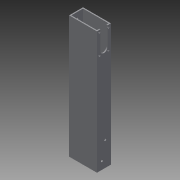
# Autodesk Inventor part: Arm_Second_Flame
Saved by Autodesk Inventor 2013 (Build 170138000, 138)
## iProperties
Created: 2014-04-16
Part Number: Arm_Second_Flame
Material: 一般
Document SubType Name: Modeling
Designer: andou
Density: 1 g/cm^3
Author: andou
Autodesk Inventor part; units mm, degrees
ref_plane "YZ Plane" through (0, 0, 0) normal (1, 0, 0) x (0, 1, 0)
ref_plane "XZ Plane" through (0, 0, 0) normal (0, 1, 0) x (-1, 0, 0)
ref_plane "XY Plane" through (0, 0, 0) normal (0, 0, 1) x (1, 0, 0)
sketch "スケッチ1" plane through (0, 0, 0) normal (0, 0, 1) x (1, 0, 0)
  line L0 (-25, 12.5) -> (25, 12.5)
  line L1 (25, 12.5) -> (25, -12.5)
  line L2 (25, -12.5) -> (-25, -12.5)
  line L3 (-25, -12.5) -> (-25, 12.5)
  line L4 (-23, 10.5) -> (23, 10.5)
  line L5 (23, 10.5) -> (23, -10.5)
  line L6 (23, -10.5) -> (-23, -10.5)
  line L7 (-23, -10.5) -> (-23, 10.5)
  point P0 (0, 0)
  dimension "d0" = 50
  dimension "d2" = 25
  dimension "d3" = 21
  dimension "d4" = 46
  dimension "d5" = 23
  dimension "d6" = 25
  dimension "d7" = 10.5
  dimension "d8" = 12.5
  constraints: 16 end point, 4 parallel, 2 horizontal, 2 perpendicular
  measures "d0" distance of L0.start L0.end
  measures "d2" distance of L2.end L0.start
  measures "d3" distance of L6.end L4.start
  measures "d4" distance of L4.start L4.end
  measures "d5" distance from line of point (0, 0) L7
  measures "d6" distance from line of point (0, 0) L1
  measures "d7" distance from line of L4 point (0, 0)
  measures "d8" distance from line of point (0, 0) L2
extrude "押し出し1" add sketch "スケッチ1" against normal blind 220
sketch "スケッチ2" plane through (25, -12.5, 0) normal (1, 0, 0) x (0, 0, -1)
  line L0 (0, 0) -> (220, 0) projected
  line L1 (220, 25) -> (220, 0) projected
  circle A0 centre (176, 15) radius 2
  circle A1 centre (206, 9) radius 2
  point P0 (0, 12.5)
  dimension "d11" = 4
  dimension "d13" = 30
  dimension "d16" = 14
  dimension "d17" = 9
  dimension "d61" = 15
  constraints: 2 centre point, 1 equal radius
  measures "d11" diameter of A0
  measures "d13" horizontal distance of A1.centre A0.centre
  measures "d16" distance from line of L1 A1.centre
  measures "d17" distance from line of L0 A1.centre
  measures "d61" distance from line of L0 A0.centre
hole "穴1" at (25, -3.5, -206) at (25, 2.5, -176) direction (-1, 0, 0) diameter 4 end through all
sketch "スケッチ3" plane through (25, -12.5, 0) normal (1, 0, 0) x (0, 0, -1)
  line L0 (0, 25) -> (0, 0) projected
  line L1 (0, 0) -> (220, 0) projected
  circle A0 centre (10.5, 12.5) radius 2
  point P0 (0, 12.5)
  dimension "d25" = 4
  dimension "d27" = 12.5
  dimension "d28" = 10.5
  constraints: 1 centre point
  measures "d25" diameter of A0
  measures "d27" distance from line of L1 A0.centre
  measures "d28" distance from line of A0.centre L0
hole "穴2" at (25, 0, -10.5) direction (-1, 0, 0) diameter 4 end through all
sketch "スケッチ4" plane through (25, -12.5, 0) normal (1, 0, 0) x (0, 0, -1)
  circle A0 centre (10.5, 12.5) radius 2 projected
  line L0 (0, 25) -> (0, 0) projected
  line L1 (0, 19) -> (33.5, 19)
  line L2 (33.5, 6) -> (0, 6)
  line L3 (0, 6) -> (0, 19)
  arc A1 (33.5, 6) -> (33.5, 19) centre (33.5, 12.5) ccw
  point P0 (0, 12.5)
  dimension "d36" = 13
  dimension "d38" = 6.5
  dimension "d39" = 13
  dimension "d40" = 33.5
  constraints: 6 end point, 2 point on circle, 1 centre point, 1 horizontal, 1 parallel, 1 point on line
  measures "d36" distance between parallel lines of L1 L2
  measures "d38" distance from line of point (0, 12.5) L2
  measures "d39" diameter of A1
  measures "d40" distance from line of L0 A1.centre
extrude "押し出し2" cut sketch "スケッチ4" against normal blind 2
sketch "スケッチ5" plane through (25, -12.5, -220) normal (1, 0, 0) x (0, 0, -1)
  arc A0 (-186.5, 6) -> (-186.5, 19) centre (-186.5, 12.5) ccw projected
  line L0 (-220, 6) -> (-220, 0) projected
  line L1 (-220, 25) -> (-220, 19) projected
  circle A1 centre (-216, 4.5) radius 1
  circle A2 centre (-216, 20.5) radius 1
  circle A3 centre (-180, 20.5) radius 1
  circle A4 centre (-180, 4.5) radius 1
  point P0 (-220, 12.5)
  dimension "d43" = 36
  dimension "d45" = 36
  dimension "d46" = 16
  dimension "d47" = 8
  dimension "d48" = 2
  dimension "d49" = 16
  dimension "d50" = 8
  dimension "d51" = 4
  dimension "d52" = 4
  constraints: 4 centre point, 3 equal radius
  measures "d43" distance of A3.centre A2.centre
  measures "d45" distance of A4.centre A1.centre
  measures "d46" distance of A2.centre A1.centre
  measures "d47" vertical distance of A1.centre point (-220, 12.5)
  measures "d48" diameter of A2
  measures "d49" distance of A4.centre A3.centre
  measures "d50" vertical distance of A0.centre A4.centre
  measures "d51" distance from line of L1 A2.centre
  measures "d52" distance from line of A1.centre L0
hole "穴3" at (25, 8, -4) at (25, -8, -4) at (25, -8, -40) at (25, 8, -40) direction (-1, 0, 0) diameter 2 depth 2.5 tip angle 118 counterbore diameter 4 counterbore depth 0.5
